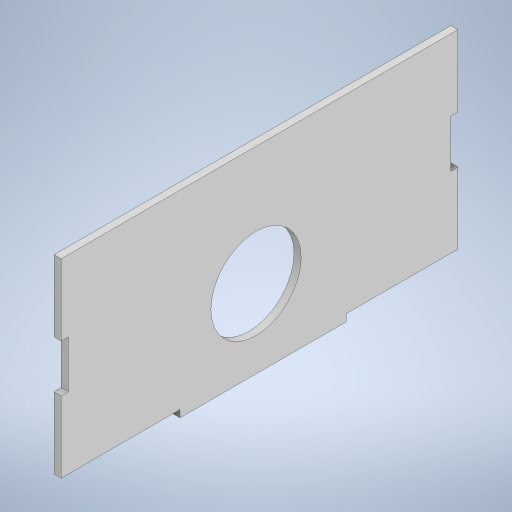
# Autodesk Inventor part: Kanan Kipas
Saved by Autodesk Inventor 2024 (Build 280153000, 153)
## iProperties
Created: 2023-08-09
Part Number: Kanan Kipas
Material: Generic
Document SubType Name: Modeling
Designer: Asus
Density: 1 g/cm^3
Appearance: Default
Author: Asus
Autodesk Inventor part; units mm, degrees
ref_plane "YZ Plane" through (0, 0, 0) normal (1, 0, 0) x (0, 1, 0)
ref_plane "XZ Plane" through (0, 0, 0) normal (0, 1, 0) x (-1, 0, 0)
ref_plane "XY Plane" through (0, 0, 0) normal (0, 0, 1) x (1, 0, 0)
sketch "Sketch2" plane through (0, 0, 0) normal (1, 0, 0) x (0, 1, 0)
  line L0 (0, 0) -> (3, 0) construction
  line L1 (3, 0) -> (3, -3)
  line L2 (3, -3) -> (3, -50)
  line L3 (3, -50) -> (0, -50)
  line L4 (0, -50) -> (0, -120)
  line L5 (0, -120) -> (3, -120)
  line L6 (3, -120) -> (3, -167)
  line L7 (3, -167) -> (33, -167)
  line L8 (33, -167) -> (33, -164)
  line L9 (33, -164) -> (53, -164)
  line L10 (53, -164) -> (53, -167)
  line L11 (53, -167) -> (83, -167)
  line L12 (83, -167) -> (83, -117)
  line L13 (83, -117) -> (83, 0)
  line L14 (83, 0) -> (53, 0)
  line L15 (53, 0) -> (53, -3)
  line L16 (53, -3) -> (33, -3)
  line L17 (33, -3) -> (33, 0)
  line L18 (33, 0) -> (3, 0)
  line L19 (0, 0) -> (0, -63) construction
  line L20 (0, -63) -> (14, -63) construction
  line L21 (14, -63) -> (14, -82) construction
  line L22 (14, -82) -> (33, -82) construction
  circle A0 centre (33, -82) radius 19
  dimension "d0" = 3
  dimension "d1" = 3
  dimension "d2" = 47
  dimension "d3" = 70
  dimension "d4" = 47
  dimension "d5" = 30
  dimension "d6" = 3
  dimension "d7" = 20
  dimension "d8" = 30
  dimension "d9" = 50
  dimension "d10" = 30
  dimension "d11" = 3
  dimension "d12" = 20
  dimension "d15" = 63
  dimension "d16" = 14
  dimension "d19" = 19
  dimension "d20" = 19
  constraints: 46 end point, 13 perpendicular, 8 point on line, 2 vertical, 1 centre point, 1 coincident, 1 horizontal
  measures "d0" distance of L0.start L0.end
  measures "d1" distance of L0.end L1.end
  measures "d2" distance of L1.end L2.end
  measures "d3" distance of L3.end L4.end
  measures "d4" distance of L5.end L6.end
  measures "d5" distance of L6.end L7.end
  measures "d6" distance of L7.end L8.end
  measures "d7" distance of L8.end L9.end
  measures "d8" distance of L10.end L11.end
  measures "d9" distance of L11.end L12.end
  measures "d10" distance of L13.end L14.end
  measures "d11" distance of L14.end L15.end
  measures "d12" distance of L15.end L16.end
  measures "d15" distance of L0.start L19.end
  measures "d16" distance of L19.end L20.end
  measures "d19" distance of L20.end L21.end
  measures "d20" distance of L21.end L22.end
extrude "Extrusion1" add sketch "Sketch2" along normal blind 3
body "Solid1"
